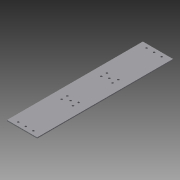
# Autodesk Inventor part: Claw Plate
Saved by Autodesk Inventor 2015 (Build 190159000, 159)
## iProperties
Created: 2015-01-25
Part Number: Claw Plate
Material: Generic
Document SubType Name: Modeling
Designer: chappelled
Density: 1 g/cm^3
Appearance: Default
Author: chappelled
Autodesk Inventor part; units mm, degrees
ref_plane "YZ Plane" through (0, 0, 0) normal (1, 0, 0) x (0, 1, 0)
ref_plane "XZ Plane" through (0, 0, 0) normal (0, 1, 0) x (-1, 0, 0)
ref_plane "XY Plane" through (0, 0, 0) normal (0, 0, 1) x (1, 0, 0)
sketch "Sketch1" plane through (0, 0, 0) normal (0, 1, 0) x (-1, 0, 0)
  line L0 (0, 0) -> (-101.6, 0)
  line L1 (-101.6, 0) -> (-101.6, 457.2)
  line L2 (-101.6, 457.2) -> (0, 457.2)
  line L3 (0, 457.2) -> (0, 0)
  point P0 (-50.8, 228.6)
  dimension "d0" = 101.6
  dimension "d1" = 457.2
  dimension "d25" = 50.8
  dimension "d26" = 228.6
  constraints: 8 end point, 2 parallel, 1 horizontal, 1 perpendicular
  measures "d0" distance of L1.end L2.end
  measures "d1" distance of L0.end L1.end
  measures "d25" distance from line of L3 point (-50.8, 228.6)
  measures "d26" distance from line of L0 point (-50.8, 228.6)
extrude "Extrusion1" add sketch "Sketch1" along normal blind 3.175
sketch "Sketch2" plane through (0, 3.175, 0) normal (0, 1, 0) x (1, 0, 0)
  line L0 (101.6, -457.2) -> (101.6, 0) projected
  line L1 (101.6, -457.2) -> (0, -457.2) projected
  line L2 (101.6, 0) -> (0, 0) projected
  point P0 (25.4, -12.7)
  point P1 (50.8, -12.7)
  point P2 (76.2, -12.7)
  point P3 (25.4, -444.5)
  point P4 (76.2, -444.5)
  point P5 (50.8, -444.5)
  dimension "d60" = 25.4
  dimension "d61" = 25.4
  dimension "d62" = 25.4
  dimension "d63" = 76.2
  dimension "d64" = 25.4
  dimension "d65" = 50.8
  dimension "d66" = 12.7
  dimension "d67" = 12.7
  dimension "d68" = 12.7
  dimension "d69" = 12.7
  dimension "d70" = 12.7
  dimension "d71" = 12.7
  measures "d60" distance of point (50.8, -12.7) point (25.4, -12.7)
  measures "d61" distance of point (76.2, -12.7) point (50.8, -12.7)
  measures "d62" distance from line of L0 point (76.2, -12.7)
  measures "d63" distance from line of L0 point (25.4, -444.5)
  measures "d64" distance from line of L0 point (76.2, -444.5)
  measures "d65" distance from line of L0 point (50.8, -444.5)
  measures "d66" distance from line of L1 point (76.2, -444.5)
  measures "d67" distance from line of L1 point (50.8, -444.5)
  measures "d68" distance from line of L1 point (25.4, -444.5)
  measures "d69" distance from line of point (50.8, -12.7) L2
  measures "d70" distance from line of L2 point (76.2, -12.7)
  measures "d71" distance from line of L2 point (25.4, -12.7)
hole "Hole6" at (25.4, 3.175, 12.7) at (50.8, 3.175, 12.7) at (76.2, 3.175, 12.7) at (25.4, 3.175, 444.5) at (76.2, 3.175, 444.5) at (50.8, 3.175, 444.5) direction (0, -1, 0) diameter 6.35 end through all
sketch "Sketch3" plane through (0, 3.175, 0) normal (0, 1, 0) x (1, 0, 0)
  line L0 (0, 0) -> (0, -457.2) projected
  line L1 (101.6, -457.2) -> (101.6, 0) projected
  line L2 (101.6, 0) -> (0, 0) projected
  line L3 (0, -228.6) -> (101.6, -228.6)
  line L4 (101.6, 0) -> (101.6, -457.2) projected
  point P0 (69.85, -152.4)
  point P1 (31.75, -152.4)
  point P2 (31.75, -171.45)
  point P3 (69.85, -171.45)
  point P4 (69.85, -152.4)
  point P5 (31.75, -304.8)
  point P6 (31.75, -285.75)
  point P7 (69.85, -285.75)
  point P8 (69.85, -304.8)
  dimension "d79" = 38.1
  dimension "d80" = 19.05
  dimension "d81" = 31.75
  dimension "d82" = 31.75
  dimension "d83" = 152.4
  dimension "d84" = 19.05
  dimension "d85" = 38.1
  dimension "d86" = 152.4
  constraints: 4 symmetric about line, 2 end point, 2 midpoint, 1 coincident
  measures "d79" distance of point (69.85, -152.4) point (31.75, -152.4)
  measures "d80" distance of point (31.75, -171.45) point (31.75, -152.4)
  measures "d81" distance from line of L0 point (31.75, -152.4)
  measures "d82" distance from line of L1 point (69.85, -171.45)
  measures "d83" distance from line of L2 point (31.75, -152.4)
  measures "d84" distance of point (69.85, -171.45) point (69.85, -152.4)
  measures "d85" distance of point (69.85, -171.45) point (31.75, -171.45)
  measures "d86" distance from line of L2 point (69.85, -152.4)
hole "Hole7" at (69.85, 3.175, 152.4) at (31.75, 3.175, 152.4) at (31.75, 3.175, 171.45) at (69.85, 3.175, 171.45) at (31.75, 3.175, 285.75) at (31.75, 3.175, 304.8) at (69.85, 3.175, 304.8) at (69.85, 3.175, 285.75) direction (0, -1, 0) diameter 6.35 end through all
sketch "Sketch4" plane through (0, 3.175, 0) normal (0, 1, 0) x (1, 0, 0)
  line L0 (0, 0) -> (0, -457.2) projected
  line L1 (101.6, 0) -> (0, 0) projected
  point P0 (50.8, -163.5125)
  point P1 (50.8, -293.6875)
  dimension "d94" = 130.175
  dimension "d95" = 50.8
  dimension "d96" = 50.8
  dimension "d97" = 163.5125
  measures "d94" distance of point (50.8, -293.688) point (50.8, -163.512)
  measures "d95" distance from line of L0 point (50.8, -163.512)
  measures "d96" distance from line of L0 point (50.8, -293.688)
  measures "d97" distance from line of point (50.8, -163.512) L1
hole "Hole8" at (50.8, 3.175, 163.5125) at (50.8, 3.175, 293.6875) direction (0, -1, 0) diameter 6.35 end through all
body "Solid1"
